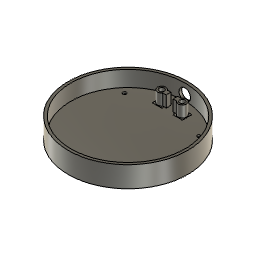
Spacemouse Compact Housing (Autodesk Fusion 360 archive; units mm, degrees)
design "Spacemouse mount" references "Spacemouse Compact 'module'"
Autodesk Fusion 360 part; units mm, degrees
derive "Sketch1" from "Spacemouse Compact 'module' v6"
sketch "sketch 195" plane through (0, 0, 0) normal (0, 0, 1) x (1, 0, 0)
  circle A0 centre (0, 0) radius 34.75
  circle A1 centre (0, -29) radius 2
  circle A2 centre (0, -29) radius 1
  circle A3 centre (0, 0) radius 33
  circle A4 centre (0, 0) radius 32.1
  line L0 (0, -30) -> (-22.5, 20.1871)
  line L1 (-22.5, 20.1871) -> (22.5, 20.1871)
  line L2 (22.5, 20.1871) -> (0, -30)
  line L3 (0, -32.45) -> (0, -25.55)
  line L4 (0, 0) -> (0, -32.45)
  circle A5 centre (-21.6606, 19.6436) radius 1
  line L5 (0.4483, -29) -> (-0.4483, -29)
  circle A6 centre (-21.6606, 19.6436) radius 2
  line L6 (-21.6606, 19.6436) -> (-24.5565, 21.5189)
  circle A7 centre (21.6606, 19.6436) radius 1
  line L7 (-21.6606, 19.6436) -> (-21.3086, 20.1871)
  line L8 (-21.6606, 19.6436) -> (-22.0126, 19.1)
  line L9 (21.6606, 19.6436) -> (24.5565, 21.5189)
  line L10 (21.6606, 19.6436) -> (21.3086, 20.1871)
  line L11 (21.6606, 19.6436) -> (22.0126, 19.1)
  circle A8 centre (21.6606, 19.6436) radius 2
  line L12 (21.6606, 19.6436) -> (18.7648, 17.7683)
extrude "Extrude1" add sketch "sketch 195" along normal blind 6.8 contours A0 makes body 1
extrude "Extrude2" add sketch "sketch 195" along normal blind 2 contours A1 A2 L2 L3 L4 | A1 A4 L2 L3 L4 L9 A8 | A1 A2 L2 L3 L4 | A1 L0 L1 L2 A6 A8 | A1 A4 L0 L3 L4 A6 L6 | A1 A2 L0 L3 L4 | A1 A2 L0 L3 L4 | L2 A7 A8 L12 | L2 A7 L9 A8 | L1 A7 A8 L12 | L0 A5 A6 L6 | L0 L1 A5 A6 | A4 L1 A6 L6 L9 A8 | L1 A7 L9 A8 | L1 A5 A6 L6 | A3 bodies 1
extrude "Extrude13" add sketch "sketch 195" against normal blind 1 contours A0 | A1 A2 L2 L3 L4 | A1 A4 L2 L3 L4 L9 A8 | A1 A2 L2 L3 L4 | A1 L0 L1 L2 A6 A8 | A1 A4 L0 L3 L4 A6 L6 | A1 A2 L0 L3 L4 | A1 A2 L0 L3 L4 | L2 A7 A8 L12 | L2 A7 L9 A8 | L1 A7 A8 L12 | L0 A5 A6 L6 | L0 L1 A5 A6 | A4 L1 A6 L6 L9 A8 | L1 A7 L9 A8 | L1 A5 A6 L6 | A3 bodies 1
extrude "Extrude3" add 1 faces at (33.9144, -3.3659, 6.8) along direction (0, 0, 1) blind 4.36 on bodies 1 bodies 1
sketch "Sketch1" plane through (0, 0, 2) normal (0, 0, 1) x (-1, 0, 0)
  line L0 (0, 0) -> (0, -34.75)
  circle A0 centre (0, 0) radius 34.5
  circle A1 centre (0, 0) radius 33
  circle A2 centre (0, 0) radius 34.75
  line L1 (0, -34.75) -> (0, -19.75)
  line L2 (0, -19.75) -> (0, -24.25)
  line L3 (0, -24.25) -> (-2, -24.25)
  line L4 (0, -24.25) -> (2, -24.25)
  line L5 (2, -24.25) -> (2, -27)
  line L6 (2, -27) -> (-2, -27)
  line L7 (-2, -27) -> (-2, -24.25)
  line L8 (0, -24.25) -> (0, -27)
  line L9 (2, -27) -> (2, -27.8611)
  line L10 (2, -24.25) -> (2, -23.3889)
  line L11 (-2, -24.25) -> (-2, -23.3889)
  line L12 (-2, -27) -> (-2, -27.8611)
  line L13 (4.5, -21.5) -> (-4.5, -29.5) construction
  line L14 (-4.5, -21.5) -> (4.5, -29.5) construction
  line L15 (2, -27) -> (8, -27)
  line L16 (-2, -27) -> (-8, -27)
  line L17 (-2, -24.25) -> (-8, -24.25)
  line L18 (-8, -24.25) -> (-8, -27)
  circle A3 centre (6, -25.625) radius 1.5
  circle A4 centre (-6, -25.625) radius 1.5
  line L19 (2, -24.25) -> (8, -24.25)
  line L20 (8, -27) -> (8, -24.25)
  circle A5 centre (21.6606, -19.6436) radius 1
  circle A6 centre (-21.6606, -19.6436) radius 1
  circle A7 centre (0, 29) radius 1
  line L21 (-2, -27) -> (-6, -27)
  line L22 (-6, -27) -> (-6, -24.25)
  circle A8 centre (-6, -25.625) radius 2.4271
  line L23 (2, -27) -> (6, -27)
  line L24 (6, -27) -> (6, -24.25)
  circle A9 centre (6, -25.625) radius 2.4271
  point P0 (0, -25.5)
  dimension "d8" = 69
  dimension "d9" = 15
  dimension "d10" = 4.5
  dimension "d11" = 2
  dimension "d12" = 2
  dimension "d13" = 2.75
  dimension "d36" = 6
  dimension "d37" = 3
  dimension "d38" = 3
  dimension "d44" = 6
  dimension "d60" = 4
  dimension "d61" = 4
  constraint coincident L0.start A0.centre
  constraint vertical L0
  constraint coincident L0.end A2
  constraint parallel L0 L1
  constraint parallel L0 L2
  constraint perpendicular L2 L3
  constraint perpendicular L0 L4
  constraint perpendicular L4 L5
  constraint perpendicular L1 L6
  constraint midpoint L6 L8.end
  constraint perpendicular L6 L9
  constraint perpendicular L4 L10
  constraint perpendicular L3 L11
  constraint perpendicular L6 L12
  constraint coincident L13 P0
  constraint coincident L14 P0
  constraint perpendicular L7 L16
  constraint perpendicular L11 L17
  constraint perpendicular L16 L18
  constraint perpendicular L19 L20
  constraint perpendicular L7 L21
  constraint coincident L17 L22.end
  constraint perpendicular L17 L22
  constraint midpoint A4.centre L22
  constraint concentric A4 A8
  constraint coincident L16.end A8
  constraint perpendicular L5 L23
  constraint coincident L19 L24.end
  constraint perpendicular L19 L24
  constraint midpoint A3.centre L24
  constraint concentric A3 A9
  constraint coincident L15.end A9
  measures "d8" diameter of A0
  measures "d9" distance of L0.end L1.end
  measures "d10" distance of L1.end L2.end
  measures "d11" distance of L2.end L3.end
  measures "d12" distance of L2.end L4.end
  measures "d13" distance of L4.end L5.end
  measures "d36" distance of L3.end L17.end
  measures "d37" diameter of A3
  measures "d38" diameter of A4
  measures "d44" distance of L4.end L19.end
  measures "d60" distance of L6.end L21.end
  measures "d61" distance of L5.end L23.end
extrude "Extrude4" add sketch "Sketch1" along normal blind 6.6 separate body contours L7 L16 L17 L21 A8 | L5 L15 L19 L23 A9 | L16 L17 A4 L21 A8 | L17 A4 A8 | A3 L19 A9 | L15 A3 L19 L23 A9 | L15 A3 L23 A9 | L16 A4 L21 A8 | L16 L17 L18 A4 | L18 A8 | L15 A3 L19 L20 | L20 A9 makes body 2 at (8.072, 24.3612, 4.2) makes body 3 at (-4.1466, 27.192, 4.2)
sketch "Sketch2" plane through (0, 24.25, 3.498) normal (0, -1, 0) x (-1, 0, 0)
  circle A0 centre (0, -1.852) radius 3.35
  line L0 (-2, 1.498) -> (-4, 1.498)
  line L1 (-4, -5.102) -> (-2, -5.102)
  line L2 (-2, -5.102) -> (-2, 1.498)
  line L3 (-2, 1.498) -> (2, 1.498)
  line L4 (0, -1.852) -> (0, 1.498)
  line L5 (4, 1.498) -> (2, 1.498)
  line L6 (2, -5.102) -> (4, -5.102)
  line L7 (-4, 1.498) -> (-4, -5.102)
  line L8 (2, 1.498) -> (2, -5.102)
  line L9 (4, -5.102) -> (4, 1.498)
  dimension "d20" = 6.7
  constraint coincident L0.start L2.end
  constraint coincident L3.end L5.end
  constraint coincident A0.centre L4.start
  constraint coincident A0 L4.end
  constraint vertical L4
  constraint midpoint L3 L4.end
  measures "d20" diameter of A0
extrude "Extrude10" cut sketch "Sketch2" along normal blind -36 and the other way blind 9 contours A0 L8 | A0 L2 L8 | A0 L2 bodies 1
ref_plane "WorkPlane2" through (3, 24.25, 5.3) normal (0, -1, 0) x (1, 0, 0)
extrude "Extrude11" cut sketch "Sketch2" along normal blind -15 and the other way blind 5 contours A0 L8 | A0 L2 L8 | A0 L2 bodies 1
sketch "Sketch4" plane through (0, 0, 2) normal (0, 0, 1) x (-1, 0, 0)
  circle A0 centre (0, 0) radius 33
  line L0 (8.75, -22.875) -> (3.25, -22.875)
  line L1 (3.25, -22.875) -> (3.25, -28.375)
  line L2 (3.25, -28.375) -> (8.75, -28.375)
  line L3 (8.75, -28.375) -> (8.75, -22.875)
  line L4 (8.75, -22.875) -> (3.25, -28.375) construction
  line L5 (3.25, -22.875) -> (8.75, -28.375) construction
  line L6 (-3.25, -22.875) -> (-8.75, -22.875)
  line L7 (-8.75, -22.875) -> (-8.75, -28.375)
  line L8 (-8.75, -28.375) -> (-3.25, -28.375)
  line L9 (-3.25, -28.375) -> (-3.25, -22.875)
  line L10 (-3.25, -22.875) -> (-8.75, -28.375) construction
  line L11 (-8.75, -22.875) -> (-3.25, -28.375) construction
  circle A1 centre (21.6606, -19.6436) radius 1
  circle A2 centre (-21.6606, -19.6436) radius 1
  circle A3 centre (0, 29) radius 1
  circle A4 centre (-6, -25.625) radius 1.5
  circle A5 centre (6, -25.625) radius 1.5
  point P0 (6, -25.625)
  point P1 (-6, -25.625)
  dimension "d45" = 5.5
  dimension "d46" = 5.5
  dimension "d47" = 5.5
  dimension "d48" = 5.5
  constraint horizontal L0
  constraint perpendicular L0 L1
  constraint parallel L0 L2
  constraint parallel L1 L3
  constraint coincident L4 P0
  constraint coincident L5 P0
  constraint coincident P0 A5.centre
  constraint horizontal L6
  constraint perpendicular L6 L7
  constraint parallel L6 L8
  constraint parallel L7 L9
  constraint coincident L10 P1
  constraint coincident L11 P1
  constraint coincident P1 A4.centre
  measures "d45" distance of L0.end L1.end
  measures "d46" distance of L1.end L2.end
  measures "d47" distance of L7.end L8.end
  measures "d48" distance of L6.end L7.end
extrude "Extrude12" cut sketch "Sketch4" against normal blind 2 contours L0 L1 L2 L3 | L6 L7 L8 L9 | A4 | A5 bodies 1
sketch "Sketch5" plane through (0, 0, -1) normal (0, 0, -1) x (1, 0, 0)
  circle A0 centre (21.6606, -19.6436) radius 1
  circle A1 centre (0, 29) radius 1
  circle A2 centre (-21.6606, -19.6436) radius 1
  circle A3 centre (0, 0) radius 34.75
  circle A4 centre (-21.6606, -19.6436) radius 2
  circle A5 centre (0, 29) radius 2
  circle A6 centre (21.6606, -19.6436) radius 2
  dimension "d54" = 4
  dimension "d55" = 4
  dimension "d56" = 4
  constraint concentric A2 A4
  constraint concentric A1 A5
  constraint concentric A0 A6
  measures "d54" diameter of A4
  measures "d55" diameter of A5
  measures "d56" diameter of A6
extrude "Extrude14" cut sketch "Sketch5" against normal blind 2 contours A4 | A5 | A6 bodies 1
move_face "OffsetFaces1" offset -0.2 1 faces at (7.572, 32.1195, 6.3126) on bodies 1
